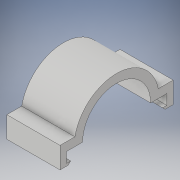
# Autodesk Inventor part: PistonClip
Saved by Autodesk Inventor 2018 (Build 220112000, 112)
## iProperties
Created: 2019-09-04
Part Number: PistonClip
Material: Generic
Document SubType Name: Modeling
Designer: 871357
Density: 1 g/cm^3
Appearance: Default
Author: 871357
Autodesk Inventor part; units mm, degrees
ref_plane "YZ Plane" through (0, 0, 0) normal (1, 0, 0) x (0, 1, 0)
ref_plane "XZ Plane" through (0, 0, 0) normal (0, 1, 0) x (-1, 0, 0)
ref_plane "XY Plane" through (0, 0, 0) normal (0, 0, 1) x (1, 0, 0)
sketch "Sketch1" plane through (0, 0, 0) normal (1, 0, 0) x (0, 1, 0)
  arc A0 (0, -20.32) -> (0, 20.32) centre (0, 0) ccw
  arc A1 (5.08, -24.8868) -> (5.08, 24.8868) centre (0, 0) ccw
  line L0 (0, 25.6032) -> (0, 20.32)
  line L1 (0, -20.32) -> (0, -25.4)
  line L2 (0, 25.6032) -> (0, 29.9668)
  line L3 (0, 29.9668) -> (-6.096, 29.9668)
  line L4 (-6.096, 29.9668) -> (-6.096, 27.4268)
  line L5 (-6.096, 27.4268) -> (-7.62, 28.9508)
  line L6 (-6.096, 27.4268) -> (-3.9407, 27.4268) construction
  line L7 (5.08, 24.8868) -> (5.08, 33.7768)
  line L8 (5.08, 33.7768) -> (-7.62, 33.7768)
  line L9 (-7.62, 33.7768) -> (-7.62, 28.9508)
  line L10 (10.0375, 0) -> (16.2196, 0) construction
  line L11 (0, -25.4) -> (0, -29.9668)
  line L12 (0, -29.9668) -> (-6.096, -29.9668)
  line L13 (-6.096, -29.9668) -> (-6.096, -27.4268)
  line L14 (-6.096, -27.4268) -> (-7.62, -28.9508)
  line L15 (5.08, -24.8868) -> (5.08, -33.7768)
  line L16 (5.08, -33.7768) -> (-7.62, -33.7768)
  line L17 (-7.62, -33.7768) -> (-7.62, -28.9508)
  dimension "d0" = 40.64
  dimension "d1" = 50.8
  dimension "d3" = 6.096
  dimension "d4" = 2.54
  dimension "d5" = 135
  dimension "d6" = 5.08
  dimension "d7" = 0
  dimension "d8" = 8.89
  dimension "d9" = 12.7
  dimension "d12" = 5.08
  constraints: 36 end point, 7 symmetric about line, 5 vertical, 4 point on circle, 3 horizontal, 2 centre point, 2 coincident, 2 perpendicular, 1 equal length
  measures "d0" diameter of A0
  measures "d1" diameter of A1
  measures "d3" distance of L2.end L3.end
  measures "d4" distance of L3.end L4.end
  measures "d5" angle of L6 L5
  measures "d6" distance between parallel lines of L2 L7
  measures "d7" distance from line of point (0, 0) L0
  measures "d8" distance of L7.start L7.end
  measures "d9" distance of L7.end L8.end
  measures "d12" distance from line of L7.start L3
extrude "Extrusion1" add sketch "Sketch1" along normal mid plane 31.75
body "Solid1"
